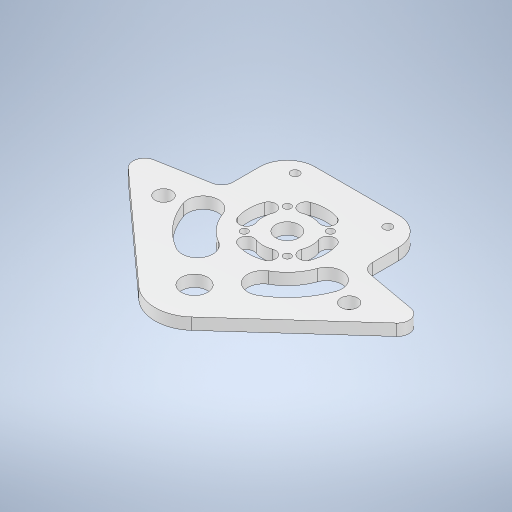
# Autodesk Inventor part: Chassis
Saved by Autodesk Inventor 2023.2 (Build 272271000, 271)
## iProperties
Created: 2022-05-26
Part Number: Chassis
Material: Aluminum 6061
Document SubType Name: Modeling
Designer: Nathan Cai
Density: 2.7 g/cm^3
Appearance: Aluminum - Flat
Mass: 52.277 g
Surface Area: 118.458 cm^2
Volume: 19.3619 cm^3
Pulley_Spacing: 1.500 in
Author: Nathan Cai
Autodesk Inventor part; units mm, degrees
ref_plane "YZ Plane" through (0, 0, 0) normal (1, 0, 0) x (0, 1, 0)
ref_plane "XZ Plane" through (0, 0, 0) normal (0, 1, 0) x (-1, 0, 0)
ref_plane "XY Plane" through (0, 0, 0) normal (0, 0, 1) x (1, 0, 0)
sketch "Sketch1" plane through (0, 0, 0) normal (0, 1, 0) x (-1, 0, 0)
  line L0 (101.6, 38.1) -> (-101.6, 38.1) construction
  line L1 (-101.6, 38.1) -> (-101.6, -38.1) construction
  line L2 (-101.6, -38.1) -> (101.6, -38.1) construction
  line L3 (101.6, -38.1) -> (101.6, 38.1) construction
  line L4 (101.6, 38.1) -> (-101.6, -38.1) construction
  line L5 (-101.6, 38.1) -> (101.6, -38.1) construction
  line L6 (-28.575, 66.675) -> (28.575, 66.675) construction
  line L7 (28.575, 66.675) -> (28.575, 9.525)
  line L8 (28.575, 9.525) -> (-28.575, 9.525)
  line L9 (-28.575, 9.525) -> (-28.575, 66.675)
  line L10 (-28.575, 66.675) -> (28.575, 9.525) construction
  line L11 (28.575, 66.675) -> (-28.575, 9.525) construction
  circle A0 centre (-38.1, 50.8) radius 3.429
  line L12 (0, 38.1) -> (0, -38.1) construction
  circle A1 centre (-38.1, 50.8) radius 9.525 construction
  line L13 (-38.1, 60.325) -> (-28.575, 60.325) construction
  circle A2 centre (38.1, 50.8) radius 3.429
  circle A3 centre (38.1, 50.8) radius 9.525 construction
  line L14 (38.1, 60.325) -> (28.575, 60.325) construction
  circle A4 centre (-76.2, -38.1) radius 1.7526
  circle A5 centre (-95.25, 3.175) radius 1.7526
  circle A6 centre (76.2, -38.1) radius 1.7526
  circle A7 centre (95.25, 3.175) radius 1.7526
  line L15 (-101.6, -38.1) -> (-101.6, 6.35)
  line L16 (-101.6, 6.35) -> (-10.8392, 88.2168)
  line L17 (101.6, -38.1) -> (101.6, 6.35)
  line L18 (101.6, 6.35) -> (10.8392, 88.2168)
  line L19 (-42.6417, 42.4275) -> (-87.975, 1.5367)
  line L20 (-87.975, 1.5367) -> (-87.975, -38.1)
  line L21 (87.975, -38.1) -> (87.975, 1.5367)
  line L22 (87.975, 1.5367) -> (42.6417, 42.4275)
  line L23 (0, -38.1) -> (-95.25, -38.1) construction
  line L24 (0, -38.1) -> (95.25, -38.1) construction
  circle A8 centre (-60.325, 35.0287) radius 1.7526
  circle A9 centre (-33.3375, 31.75) radius 1.7526
  line L25 (-38.1, 0) -> (-38.1, 41.275)
  line L26 (-38.1, 0) -> (0, 0) construction
  circle A10 centre (60.325, 35.0287) radius 1.7526
  circle A11 centre (33.3375, 31.75) radius 1.7526
  line L27 (38.1, 0) -> (38.1, 41.275)
  line L28 (38.1, 0) -> (0, 0) construction
  line L29 (-87.975, 0) -> (-65.115, 0)
  line L30 (-65.115, 0) -> (-65.115, -31.75)
  line L31 (-65.115, -31.75) -> (-87.975, -31.75)
  line L32 (-101.6, -38.1) -> (101.6, -38.1) construction
  line L33 (101.6, -38.1) -> (101.6, 19.05)
  line L34 (101.6, 19.05) -> (-101.6, 19.05) construction
  line L35 (-101.6, 19.05) -> (-101.6, -38.1)
  line L36 (-101.6, 19.05) -> (-87.5203, 19.05) construction
  line L37 (87.5203, 19.05) -> (101.6, 19.05) construction
  circle A12 centre (-38.1, 0) radius 3.175 construction
  circle A13 centre (-38.1, 0) radius 6.35 construction
  circle A14 centre (38.1, 0) radius 3.175 construction
  circle A15 centre (38.1, 0) radius 6.35 construction
  circle A16 centre (28.575, 9.525) radius 1.7526
  circle A17 centre (28.575, 9.525) radius 4.7625
  arc A18 (17.0773, 9.525) -> (28.575, 21.0227) centre (17.0773, 21.0227) ccw
  circle A19 centre (-28.575, 9.525) radius 1.7526
  circle A20 centre (-28.575, 9.525) radius 4.7625
  arc A21 (-28.575, 21.0227) -> (-17.0773, 9.525) centre (-17.0773, 21.0227) ccw
  arc A22 (31.4325, 5.715) -> (38.1, 19.05) centre (21.4312, 19.05) ccw
  arc A23 (-38.1, 19.05) -> (-31.4325, 5.715) centre (-21.4312, 19.05) ccw
  line L38 (-61.94, -38.1) -> (-61.94, 25.0204)
  line L39 (87.975, 0) -> (65.115, 0)
  line L40 (65.115, 0) -> (65.115, -31.75)
  line L41 (65.115, -31.75) -> (87.975, -31.75)
  line L42 (61.94, -38.1) -> (61.94, 25.0204)
  line L43 (-28.575, 4.7625) -> (28.575, 4.7625)
  line L44 (101.6, -31.75) -> (-101.6, -31.75)
  line L45 (-101.6, -31.75) -> (-101.6, -44.45) construction
  line L46 (-101.6, -44.45) -> (101.6, -44.45)
  line L47 (101.6, -44.45) -> (101.6, -31.75) construction
  circle A24 centre (0, -38.1) radius 1.7526
  circle A25 centre (38.1, -38.1) radius 1.7526
  circle A26 centre (-38.1, -38.1) radius 1.7526
  line L48 (101.6, -38.1) -> (76.2, -44.45)
  line L49 (-101.6, -38.1) -> (-76.2, -44.45)
  line L50 (76.2, -38.1) -> (76.2, -44.45) construction
  line L51 (-76.2, -38.1) -> (-76.2, -44.45) construction
  line L52 (59.1924, 41.2769) -> (32.488, 36.4361)
  circle A27 centre (60.325, 35.0287) radius 6.35
  circle A28 centre (33.3375, 31.75) radius 4.7625
  line L53 (-59.1924, 41.2769) -> (-32.488, 36.4361)
  circle A29 centre (-60.325, 35.0287) radius 6.35
  circle A30 centre (-33.3375, 31.75) radius 4.7625
  line L54 (-87.975, 0) -> (-65.115, 0)
  line L55 (-65.115, 0) -> (-65.115, -3.175)
  line L56 (-65.115, -3.175) -> (-87.975, -3.175)
  line L57 (-87.975, -3.175) -> (-87.975, 0)
  line L58 (-65.115, -15.875) -> (-87.975, -15.875) construction
  line L59 (-65.115, -28.575) -> (-87.975, -28.575)
  line L60 (-84.8, -38.1) -> (-84.8, 0.1248)
  line L61 (65.115, -3.175) -> (87.975, -3.175)
  line L62 (65.115, -15.875) -> (87.975, -15.875) construction
  line L63 (65.115, -28.575) -> (87.975, -28.575)
  line L64 (84.8, -38.1) -> (84.8, 0.1248)
  circle A31 centre (0, 38.1) radius 22.225 construction
  circle A32 centre (0, 38.1) radius 12.5 construction
  circle A33 centre (8.8388, 46.9388) radius 1.5
  circle A34 centre (-8.8388, 46.9388) radius 1.5
  circle A35 centre (-8.8388, 29.2612) radius 1.5
  circle A36 centre (8.8388, 29.2612) radius 1.5
  circle A37 centre (0, 38.1) radius 4.7625
  circle A38 centre (-19.05, 15.875) radius 1.7526
  circle A39 centre (19.05, 15.875) radius 1.7526
  arc A40 (4.4463, 50.316) -> (-4.4463, 50.316) centre (0, 38.1) ccw construction
  arc A41 (5.4723, 53.1351) -> (-5.4723, 53.1351) centre (0, 38.1) ccw
  arc A42 (3.4202, 47.4969) -> (-3.4202, 47.4969) centre (0, 38.1) ccw
  arc A43 (3.4202, 47.4969) -> (5.4723, 53.1351) centre (4.4463, 50.316) ccw
  arc A44 (-5.4723, 53.1351) -> (-3.4202, 47.4969) centre (-4.4463, 50.316) ccw
  line L65 (0, 38.1) -> (4.4463, 50.316) construction
  line L66 (0, 38.1) -> (-4.4463, 50.316) construction
  arc A45 (-9.3969, 41.5202) -> (-15.0351, 43.5723) centre (-12.216, 42.5463) ccw
  arc A46 (-15.0351, 43.5723) -> (-15.0351, 32.6277) centre (0, 38.1) ccw
  arc A47 (-15.0351, 32.6277) -> (-9.3969, 34.6798) centre (-12.216, 33.6537) ccw
  arc A48 (-9.3969, 41.5202) -> (-9.3969, 34.6798) centre (0, 38.1) ccw
  arc A49 (-3.4202, 28.7031) -> (-5.4723, 23.0649) centre (-4.4463, 25.884) ccw
  arc A50 (-5.4723, 23.0649) -> (5.4723, 23.0649) centre (0, 38.1) ccw
  arc A51 (5.4723, 23.0649) -> (3.4202, 28.7031) centre (4.4463, 25.884) ccw
  arc A52 (-3.4202, 28.7031) -> (3.4202, 28.7031) centre (0, 38.1) ccw
  arc A53 (9.3969, 34.6798) -> (15.0351, 32.6277) centre (12.216, 33.6537) ccw
  arc A54 (15.0351, 32.6277) -> (15.0351, 43.5723) centre (0, 38.1) ccw
  arc A55 (15.0351, 43.5723) -> (9.3969, 41.5202) centre (12.216, 42.5463) ccw
  arc A56 (9.3969, 34.6798) -> (9.3969, 41.5202) centre (0, 38.1) ccw
  arc A57 (-55.063, 48.3266) -> (-52.7226, 40.1041) centre (-51.8731, 44.7902) ccw
  arc A58 (52.7226, 40.1041) -> (55.063, 48.3266) centre (51.8731, 44.7902) ccw
  circle A59 centre (0, 76.2) radius 5.3975
  circle A60 centre (0, 76.2) radius 16.183
  arc A61 (-13.4938, 61.4719) -> (-25.36, 47.3303) centre (0, 38.1) ccw construction
  arc A62 (-16.6688, 66.9711) -> (-31.327, 49.5021) centre (0, 38.1) ccw
  arc A63 (-10.3188, 55.9726) -> (-19.3929, 45.1584) centre (0, 38.1) ccw
  arc A64 (-10.3188, 55.9726) -> (-16.6688, 66.9711) centre (-13.4938, 61.4719) ccw
  arc A65 (-31.327, 49.5021) -> (-19.3929, 45.1584) centre (-25.36, 47.3303) ccw
  line L67 (0, 38.1) -> (-13.4938, 61.4719) construction
  line L68 (0, 38.1) -> (-25.36, 47.3303) construction
  arc A66 (31.327, 49.5021) -> (16.6688, 66.9711) centre (0, 38.1) ccw
  arc A67 (19.3929, 45.1584) -> (10.3188, 55.9726) centre (0, 38.1) ccw
  arc A68 (16.6688, 66.9711) -> (10.3188, 55.9726) centre (13.4938, 61.4719) ccw
  arc A69 (19.3929, 45.1584) -> (31.327, 49.5021) centre (25.36, 47.3303) ccw
  point P0 (28.575, 38.1)
  point P1 (-28.575, 38.1)
  point P2 (28.575, 60.325)
  point P3 (-44.4797, 57.8728)
  point P4 (44.4797, 57.8728)
  point P5 (44.4797, 57.8728)
  point P6 (101.6, -15.875)
  point P7 (38.1, 41.275)
  point P8 (-87.975, -31.75)
  point P9 (-101.6, 6.35)
  point P10 (101.6, 6.35)
  point P11 (31.75, 0)
  point P12 (38.1, 6.35)
  point P13 (-38.1, 6.35)
  point P14 (-31.75, 0)
  point P15 (87.975, 0)
  point P16 (61.94, 25.0204)
  point P17 (-17.0773, 9.525)
  point P18 (-28.575, 21.0227)
  point P19 (-38.1, 19.05)
  point P20 (-31.4325, 5.715)
  point P21 (-21.8502, 0)
  point P22 (21.8502, 0)
  point P23 (-25.2074, 12.8926)
  point P24 (-28.575, 14.2875)
  point P25 (-23.8125, 9.525)
  point P26 (-28.575, 50.8)
  point P27 (25.2074, 12.8926)
  point P28 (28.575, 14.2875)
  point P29 (23.8125, 9.525)
  point P30 (28.575, 50.8)
  point P31 (26.8224, 9.525)
  point P32 (28.575, 11.2776)
  point P33 (61.94, -31.75)
  point P34 (-61.94, -31.75)
  point P35 (-28.575, 31.75)
  point P36 (-64.5781, 39.7439)
  point P37 (64.5781, 39.7439)
  point P38 (28.575, 31.75)
  point P39 (-84.8, -3.175)
  point P40 (-84.8, -28.575)
  point P41 (84.8, -3.175)
  point P42 (84.8, -28.575)
  point P43 (-101.6, -31.75)
  point P44 (-56.0719, 30.3135)
  point P45 (56.0719, 30.3135)
  point P46 (46.4735, 38.9713)
  point P47 (-46.4735, 38.9713)
  point P48 (-28.575, 11.2776)
  point P49 (-26.8224, 9.525)
  point P50 (55.063, 48.3266)
  dimension "d2" = 4.7625
  dimension "d3" = 0
  dimension "d134" = 25
  dimension "d0" = 203.2
  dimension "d1" = 76.2
  dimension "d4" = 57.15
  dimension "d6" = 6.858
  dimension "d7" = 38.1
  dimension "d8" = 19.05
  dimension "d10" = 3.5052
  dimension "d11" = 3.5052
  dimension "d12" = 0
  dimension "d14" = 25.4
  dimension "d15" = 6.35
  dimension "d20" = 50.8
  dimension "d21" = 41.275
  dimension "d22" = 44.45
  dimension "d24" = 12.7
  dimension "d25" = 13.625
  dimension "d26" = 12.7
  dimension "d27" = 13.625
  dimension "d31" = 3.5052
  dimension "d32" = 3.5052
  dimension "d33" = 6.35
  dimension "d34" = 31.75
  dimension "d35" = 4.7625
  dimension "d36" = 22.225
  dimension "d37" = 9.525
  dimension "d39" = 31.75
  dimension "d40" = 6.35
  dimension "d42" = 57.15
  dimension "d43" = 6.35
  dimension "d44" = 9.525
  dimension "d45" = 9.525
  dimension "d46" = 12.7
  dimension "d104" = 3.5052
  dimension "d105" = 9.525
  dimension "d106" = 3.175
  dimension "d107" = 22.86
  dimension "d123" = 88.9
  dimension "d124" = 12.7
  dimension "d125" = 3.5052
  dimension "d126" = 3.5052
  dimension "d127" = 38.1
  dimension "d128" = 28.575
  dimension "d129" = 3.175
  dimension "d130" = 3.175
  dimension "d133" = 44.45
  dimension "d135" = 3
  dimension "d138" = 360
  dimension "d140" = 9.525
  dimension "d141" = 3.5052
  dimension "d142" = 19.05
  dimension "d143" = 34.925
  dimension "d144" = 13
  dimension "d146" = 6
  dimension "d147" = 25
  dimension "d148" = 25
  dimension "d151" = 360
  dimension "d153" = 9.525
  dimension "d154" = 10.795
  dimension "Pulley_Spacing" = 38.1
  dimension "d157" = 26.9875
  dimension "d158" = 40
  dimension "d159" = 12.7
  dimension "d160" = 20
  constraints: 139 end point, 74 point on circle, 64 centre point, 54 symmetric about line, 30 point on line, 19 tangent, 15 coincident, 14 parallel, 9 horizontal, 9 midpoint, 9 perpendicular, 5 vertical, 1 collinear, 94 other
  measures "d0" distance of L2.end L1.end
  measures "d1" distance between parallel lines of L0 L2
  measures "d4" distance of L7.end L8.end
  measures "d6" diameter of A0
  measures "d7" distance from line of L12 A0.centre
  measures "d8" diameter of A1
  measures "d10" diameter of A4
  measures "d11" diameter of A5
  measures "d12" distance from line of L2 L51.start
  measures "d14" distance from line of L1 L51.start
  measures "d15" distance from line of L1 A5.centre
  measures "d20" distance between parallel lines of L8 L14
  measures "d21" vertical distance of L51.start A5.centre
  measures "d22" distance of L1.end L15.end
  measures "d24" distance between parallel lines of L16 L19
  measures "d25" distance between parallel lines of L15 L20
  measures "d26" distance between parallel lines of L18 L22
  measures "d27" distance from line of point (101.6, -15.875) L21
  measures "d31" diameter of A8
  measures "d32" diameter of A9
  measures "d33" distance from line of L16 A8.centre
  measures "d34" distance from line of L9 A8.centre
  measures "d35" distance from line of L9 A9.centre
  measures "d36" distance from line of L8 A9.centre
  measures "d37" distance between parallel lines of L9 L25
  measures "d39" distance between parallel lines of L31 L29
  measures "d40" distance between parallel lines of L23 L31
  measures "d42" distance of L33.end L32.end
  measures "d43" diameter of A12
  measures "d44" distance from line of L8 A12.centre
  measures "d45" distance from line of L9 A12.centre
  measures "d46" diameter of A13
  measures "d104" diameter of A16
  measures "d105" diameter of A17
  measures "d106" distance between parallel lines of L30 L38
  measures "d107" distance between parallel lines of L20 L30
  measures "d123" distance from line of L32 A1.centre
  measures "d124" distance between parallel lines of L44 L46
  measures "d125" diameter of A24
  measures "d126" diameter of A25
  measures "d127" distance of A24.centre A25.centre
  measures "d128" distance from line of L12 A16.centre
  measures "d129" distance between parallel lines of L29 L56
  measures "d130" distance between parallel lines of L20 L60
  measures "d133" diameter of A31
  measures "d135" diameter of A33
  measures "d140" diameter of A37
  measures "d141" diameter of A38
  measures "d142" horizontal distance of A1.centre A38.centre
  measures "d143" vertical distance of A1.centre A38.centre
  measures "d144" radius of A40
  measures "d146" diameter of A43
  measures "d147" angle of L10 L66
  measures "d148" angle of L11 L65
  measures "d153" diameter of A57
  measures "d154" diameter of A59
  measures "Pulley_Spacing" distance of A37.centre A59.centre
  measures "d157" radius of A61
  measures "d158" angle of L67 L68
  measures "d159" diameter of A64
  measures "d160" angle of L0 L68
extrude "Extrusion1" add sketch "Sketch1" along normal blind 4.7625 contours A66 A68 A60 L18 A58 L52 A28 L7 A69 | L7 A18 L8 A21 L9 A65 A63 A64 A60 A68 A67 A69 | A68 A60 A64 | A64 A62 A65 L9 A30 L53 A57 L16 A60
equation "\"d35\" = 0.5 * d37"
body "Solid1"
